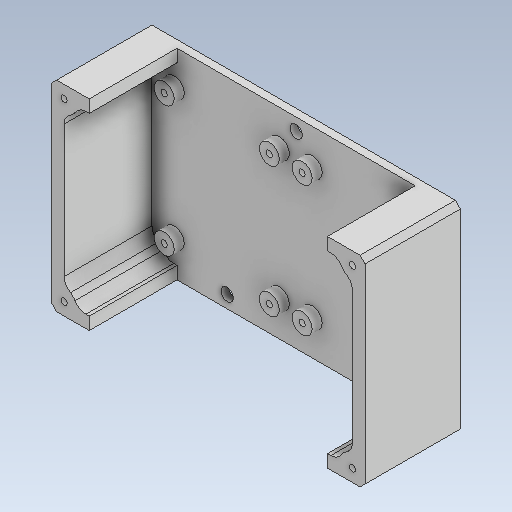
# Autodesk Inventor part: 10-06-014
Saved by Autodesk Inventor 2020 (Build 240168000, 168)
## iProperties
Created: 2020-01-11
Part Number: 10-06-014
Material: Generic
Document SubType Name: Modeling
Designer: iuliu
Density: 1 g/cm^3
Appearance: Default
Description: Cutie mofset
Mass: 68.42 g
Surface Area: 374.873 cm^2
Volume: 68.42 cm^3
Author: iuliu
Subject: 028
Autodesk Inventor part; units mm, degrees
ref_plane "YZ Plane" through (0, 0, 0) normal (1, 0, 0) x (0, 1, 0)
ref_plane "XZ Plane" through (0, 0, 0) normal (0, 1, 0) x (-1, 0, 0)
ref_plane "XY Plane" through (0, 0, 0) normal (0, 0, 1) x (1, 0, 0)
sketch "Sketch1" plane through (0, 0, 0) normal (0, 0, 1) x (1, 0, 0)
  line L0 (-62.5, 40) -> (62.5, 40)
  line L1 (62.5, 40) -> (62.5, -40)
  line L2 (62.5, -40) -> (-62.5, -40)
  line L3 (-62.5, -40) -> (-62.5, 40)
  point P0 (0, 0)
  point P1 (0, 40)
  point P2 (-62.5, 0)
  dimension "d0" = 125
  dimension "d1" = 80
  constraints: 8 end point, 2 midpoint, 2 parallel, 1 horizontal, 1 horizontal alignment, 1 perpendicular, 1 vertical alignment
  measures "d0" distance of L0.start L0.end
  measures "d1" distance of L2.end L0.start
extrude "Extrusion1" add sketch "Sketch1" along normal blind 3
sketch "Sketch2" plane through (0, 0, 3) normal (0, 0, 1) x (1, 0, 0)
  line L0 (62.5, 40) -> (-62.5, 40) projected
  line L1 (-62.5, 40) -> (-62.5, -40) projected
  line L2 (-62.5, -40) -> (62.5, -40) projected
  line L3 (62.5, -40) -> (62.5, 40) projected
  line L4 (57.5, -35) -> (-57.5, -35)
  line L5 (-57.5, -35) -> (-57.5, 35)
  line L6 (-57.5, 35) -> (57.5, 35)
  line L7 (57.5, 35) -> (57.5, -35)
  point P0 (0, 0)
  dimension "d4" = 5
  constraints: 8 end point, 3 other
  measures "d4" distance between parallel lines of L2 L4
extrude "Extrusion2" add sketch "Sketch2" along normal blind 35
sketch "Sketch3" plane through (-62.5, 40, 0) normal (0, 1, 0) x (1, 0, 0)
  line L0 (110, -38) -> (15, -38)
  line L1 (15, -38) -> (15, -3)
  line L2 (15, -3) -> (110, -3)
  line L3 (110, -3) -> (110, -38)
  line L4 (125, 0) -> (0, 0) projected
  line L5 (125, 0) -> (125, -38) projected
  line L6 (0, 0) -> (0, -38) projected
  line L7 (125, -38) -> (0, -38) projected
  point P0 (62.5, 0)
  dimension "d7" = 3
  dimension "d8" = 15
  dimension "d9" = 15
  constraints: 8 end point, 2 parallel, 1 collinear, 1 horizontal, 1 perpendicular
  measures "d7" distance between parallel lines of L4 L2
  measures "d8" distance between parallel lines of L5 L3
  measures "d9" distance between parallel lines of L6 L1
extrude "Extrusion3" cut sketch "Sketch3" against normal through all contours L0 L1 L2 L3
sketch "Sketch4" plane through (0, 0, 3) normal (0, 0, 1) x (1, 0, 0)
  circle A0 centre (57.5, -35) radius 1.25
  circle A1 centre (-57.5, -35) radius 1.25
  circle A2 centre (57.5, 35) radius 1.25
  circle A3 centre (-57.5, 35) radius 1.25
  line L0 (-62.5, 40) -> (-62.5, -40) projected
  line L1 (-47.5, 40) -> (-62.5, 40) projected
  line L2 (62.5, 40) -> (47.5, 40) projected
  line L3 (62.5, -40) -> (62.5, 40) projected
  line L4 (47.5, -40) -> (62.5, -40) projected
  line L5 (-62.5, -40) -> (-47.5, -40) projected
  point P0 (0, 0)
  dimension "d12" = 2.5
  dimension "d13" = 2.5
  dimension "d14" = 5
  dimension "d15" = 5
  dimension "d16" = 5
  dimension "d17" = 5
  dimension "d18" = 5
  dimension "d19" = 5
  dimension "d20" = 5
  dimension "d21" = 5
  constraints: 4 centre point, 2 equal radius
  measures "d12" diameter of A0
  measures "d13" diameter of A1
  measures "d14" distance from line of L0 A3.centre
  measures "d15" distance from line of L1 A3.centre
  measures "d16" distance from line of L2 A2.centre
  measures "d17" distance from line of L3 A2.centre
  measures "d18" distance from line of L3 A0.centre
  measures "d19" distance from line of A0.centre L4
  measures "d20" distance from line of L0 A1.centre
  measures "d21" distance from line of L5 A1.centre
extrude "Extrusion4" cut sketch "Sketch4" against normal through all both and the other way through all
sketch "Sketch5" plane through (0, 0, 38) normal (0, 0, 1) x (1, 0, 0)
  circle A0 centre (57.5, 35) radius 5
  circle A1 centre (57.5, -35) radius 5
  circle A2 centre (-57.5, -35) radius 5
  circle A3 centre (-57.5, 35) radius 5
  arc A4 (-56.25, 35) -> (-57.5, 33.75) centre (-57.5, 35) ccw projected
  arc A5 (-57.5, -33.75) -> (-56.25, -35) centre (-57.5, -35) ccw projected
  arc A6 (56.25, -35) -> (57.5, -33.75) centre (57.5, -35) ccw projected
  arc A7 (57.5, 33.75) -> (56.25, 35) centre (57.5, 35) ccw projected
  line L0 (62.5, -40) -> (62.5, 40) projected
  line L1 (-62.5, 40) -> (-62.5, -40) projected
  line L2 (-62.5, -40) -> (-47.5, -40) projected
  line L3 (47.5, -40) -> (62.5, -40) projected
  circle A8 centre (-57.5, -35) radius 1.25
  circle A9 centre (-57.5, 35) radius 1.25
  circle A10 centre (57.5, 35) radius 1.25
  circle A11 centre (57.5, -35) radius 1.25
  point P0 (0, 0)
  constraints: 8 centre point, 8 concentric, 4 coincident, 4 tangent
extrude "Extrusion5" add sketch "Sketch5" against normal through all contours A0 | A1 | A2 | A3
fillet "Fillet1" radius 5 8 edges at (57.5, 30, 20.5) (52.5, 35, 20.5) (52.5, -35, 20.5) (57.5, -30, 20.5) (-57.5, -30, 20.5) (-52.5, -35, 20.5) (-52.5, 35, 20.5) (-57.5, 30, 20.5)
sketch "Sketch6" plane through (0, 0, 3) normal (0, 0, 1) x (1, 0, 0)
  circle A0 centre (48.3, -25.95) radius 1.7505 construction
  circle A1 centre (6.4, -25.95) radius 1.751 construction
  circle A2 centre (-6.7, -25.95) radius 1.7505 construction
  circle A3 centre (-48.6, -25.95) radius 1.751 construction
  circle A4 centre (-48.602, 25.9501) radius 1.7529 construction
  circle A5 centre (-6.7, 25.95) radius 1.7512 construction
  circle A6 centre (48.3, 25.95) radius 1.7512 construction
  circle A7 centre (6.398, 25.9501) radius 1.7529 construction
  point P0 (0, 0)
hole "Hole1" at (-48.6, -25.95, 3) at (-48.602, 25.9501, 3) at (-6.7, 25.95, 3) at (6.398, 25.9501, 3) at (48.3, 25.95, 3) at (48.3, -25.95, 3) at (6.4, -25.95, 3) at (-6.7, -25.95, 3) direction (0, 0, -1) diameter 2.5 end through all
sketch "Sketch7" plane through (0, 0, 3) normal (0, 0, 1) x (1, 0, 0)
  circle A0 centre (6.4, -25.95) radius 1.25 projected
  circle A1 centre (48.3, 25.95) radius 1.25 projected
  circle A2 centre (-6.7, 25.95) radius 1.25 projected
  circle A3 centre (-48.6, -25.95) radius 1.25 projected
  circle A4 centre (-48.602, 25.9501) radius 1.25 projected
  circle A5 centre (6.398, 25.9501) radius 1.25 projected
  circle A6 centre (48.3, -25.95) radius 1.25 projected
  circle A7 centre (-6.7, -25.95) radius 1.25 projected
  arc A8 (-55, 30.6699) -> (-57.5, 26.3397) centre (-52.5, 26.3397) ccw projected
  line L0 (-57.5, 26.3397) -> (-57.5, -26.3397) projected
  arc A9 (-57.5, -26.3397) -> (-55, -30.6699) centre (-52.5, -26.3397) ccw projected
  arc A10 (-53.1699, -32.5) -> (-55, -30.6699) centre (-57.5, -35) ccw projected
  arc A11 (-53.1699, -32.5) -> (-48.8397, -35) centre (-48.8397, -30) ccw projected
  line L1 (-48.8397, -35) -> (-47.5, -35) projected
  line L2 (-47.5, -35) -> (-47.5, -40) projected
  line L3 (47.5, -40) -> (-47.5, -40) projected
  line L4 (47.5, -35) -> (47.5, -40) projected
  line L5 (47.5, -35) -> (48.8397, -35) projected
  arc A12 (48.8397, -35) -> (53.1699, -32.5) centre (48.8397, -30) ccw projected
  arc A13 (55, -30.6699) -> (53.1699, -32.5) centre (57.5, -35) ccw projected
  arc A14 (55, -30.6699) -> (57.5, -26.3397) centre (52.5, -26.3397) ccw projected
  line L6 (57.5, -26.3397) -> (57.5, 26.3397) projected
  arc A15 (57.5, 26.3397) -> (55, 30.6699) centre (52.5, 26.3397) ccw projected
  arc A16 (53.1699, 32.5) -> (55, 30.6699) centre (57.5, 35) ccw projected
  arc A17 (53.1699, 32.5) -> (48.8397, 35) centre (48.8397, 30) ccw projected
  line L7 (48.8397, 35) -> (47.5, 35) projected
  line L8 (47.5, 40) -> (47.5, 35) projected
  line L9 (-47.5, 40) -> (47.5, 40) projected
  line L10 (-47.5, 40) -> (-47.5, 35) projected
  line L11 (-47.5, 35) -> (-48.8397, 35) projected
  arc A18 (-48.8397, 35) -> (-53.1699, 32.5) centre (-48.8397, 30) ccw projected
  arc A19 (-55, 30.6699) -> (-53.1699, 32.5) centre (-57.5, 35) ccw projected
  circle A20 centre (48.3, -25.95) radius 4
  circle A21 centre (6.4, -25.95) radius 1.25 projected
  circle A22 centre (6.4, -25.95) radius 4
  circle A23 centre (-6.7, -25.95) radius 4
  circle A24 centre (-48.6, -25.95) radius 4
  circle A25 centre (-48.602, 25.9501) radius 4
  circle A26 centre (-6.7, 25.95) radius 4
  circle A27 centre (6.398, 25.9501) radius 4
  circle A28 centre (48.3, 25.95) radius 4
  point P0 (0, 0)
  dimension "d34" = 8
  constraints: 8 centre point, 7 coincident, 7 equal radius, 1 concentric
  measures "d34" diameter of A20
extrude "Extrusion6" add sketch "Sketch7" along normal blind 4 contours A20 | A22 | A23 | A24 | A25 | A26 | A27 | A28
chamfer "Chamfer1" distance 2 angle 45 4 edges at (-62.5, -40, 19) (-62.5, 40, 19) (62.5, -40, 19) (62.5, 40, 19)
sketch "Sketch8" plane through (0, 0, 3) normal (0, 0, 1) x (1, 0, 0)
  line L0 (47.5, -35) -> (47.5, -40) projected
  line L1 (-47.5, -40) -> (-47.5, -35) projected
  line L2 (47.5, -40) -> (-47.5, -40) projected
  line L3 (-47.5, 40) -> (47.5, 40) projected
  point P0 (0, 0)
  point P1 (27.5, -35)
  point P2 (-27.5, -35)
  point P3 (0, 35)
  point P4 (0, 40)
  dimension "d40" = 20
  dimension "d41" = 20
  dimension "d42" = 5
  dimension "d50" = 5
  constraints: 1 horizontal alignment, 1 midpoint, 1 vertical alignment
  measures "d40" distance from line of L0 point (27.5, -35)
  measures "d41" distance from line of L1 point (-27.5, -35)
  measures "d42" distance from line of point (27.5, -35) L2
  measures "d50" distance from line of L3 point (0, 35)
hole "Hole2" at (27.5, -35, 3) at (-27.5, -35, 3) at (0, 35, 3) direction (0, 0, -1) diameter 5 end through all
equation "\"d9\" = d8"
equation "\"d16\" = d15"
equation "\"d17\" = d14"
equation "\"d18\" = d17"
equation "\"d19\" = d16"
equation "\"d20\" = d19"
equation "\"d21\" = d19"
equation "\"d50\" = d42"
body "Solid1"
